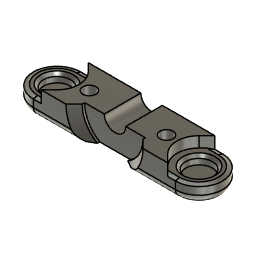
Folding propeller hub v7 (Autodesk Fusion 360 design; units mm, degrees)
Autodesk Fusion 360 part; units mm, degrees
sketch "Sketch1" plane through (0, 0, 0) normal (0, 0, 1) x (1, 0, 0)
  line L0 (-17.5, 0) -> (17.5, 0) construction
  circle A0 centre (-17.5, 0) radius 3.3
  circle A1 centre (17.5, 0) radius 3.3
  arc A2 (-17.5, 5.8) -> (-17.5, -5.8) centre (-17.5, 0) ccw
  line L1 (0, 5.8) -> (0, -5.8) construction
  arc A3 (17.5, -5.8) -> (17.5, 5.8) centre (17.5, 0) ccw
  circle A4 centre (-17.5, 0) radius 5.45
  line L2 (-17.5, 5.8) -> (17.5, 5.8)
  line L3 (17.5, -5.8) -> (-17.5, -5.8)
  line L4 (-13.6463, 3.8537) -> (-15.5925, 5.8)
  line L5 (-13.6463, -3.8537) -> (-15.5925, -5.8)
  line L6 (13.6463, 3.8537) -> (15.5925, 5.8)
  circle A5 centre (17.5, 0) radius 5.45
  line L7 (-2.5, 5.8) -> (-2.5, -5.8) construction
  line L8 (2.5, 5.8) -> (2.5, -5.8) construction
  circle A6 centre (-9.5, 0) radius 1.625
  circle A7 centre (9.5, 0) radius 1.625
  line L9 (13.6463, -3.8537) -> (15.5925, -5.8)
  dimension "d1" = 6.6
  dimension "d2" = 35
  dimension "d3" = 2.5
  dimension "d4" = 10.9
  dimension "d5" = 45
  dimension "d6" = 5
  dimension "d7" = 3.25
  dimension "d8" = 19
  dimension "d33" = 45
  constraint horizontal L0
  constraint midpoint origin L0
  constraint coincident L0.start A0.centre
  constraint coincident L0.end A1.centre
  constraint equal A0 A1
  constraint perpendicular L0 L1
  constraint symmetric A2 L1 A3
  constraint coincident origin L1
  constraint concentric A0 A4
  constraint tangent A3 L2
  constraint tangent A2 L2
  constraint tangent A2 L3
  constraint tangent A3 L3
  constraint midpoint L1.start L2
  constraint midpoint L1.end L3
  constraint coincident A4 L4.start
  constraint coincident L2 L4.end
  constraint tangent A4 L4
  constraint coincident A4 L5.start
  constraint coincident L3 L5.end
  constraint symmetric L1 A4 A5
  constraint symmetric L1 L4.start L6.start
  constraint symmetric L1 L4.end L6.end
  constraint coincident L2 L7.start
  constraint coincident L3 L7.end
  constraint perpendicular L3 L7
  constraint coincident L2 L8.start
  constraint coincident L3 L8.end
  constraint perpendicular L3 L8
  constraint coincident L0 A6.centre
  constraint coincident L0 A7.centre
  constraint symmetric L1 A6 A7
  constraint tangent A4 L5
  constraint symmetric L1 L5.start L9.start
  constraint symmetric L1 L5.end L9.end
  measures "d1" diameter of A0
  measures "d2" distance of L0.start L0.end
  measures "d3" distance of A0 A2
  measures "d4" diameter of A4
  measures "d5" angle of L2 L4
  measures "d6" distance of L7 L8
  measures "d7" diameter of A6
  measures "d8" distance of A6.centre A7.centre
  measures "d33" angle of L3 L5
extrude "Extrude1" add sketch "Sketch1" along normal mid plane 13 contours A0 | A1 | A2 A4 L2 L3 L4 L5 | A4 L2 L3 L4 L5 L6 A5 L9 | A3 L2 L3 L6 A5 L9 | A4 | A5 makes body 1
extrude "Extrude2" cut sketch "Sketch1" along normal mid plane 5.25 contours A0 | A1 | A2 A4 L2 L3 L4 L5 | A3 L2 L3 L6 A5 L9 | A4 | A5 bodies 1
extrude "Extrude3" cut sketch "Sketch1" along normal mid plane 9.4 contours A0 | A1 bodies 1
chamfer "Chamfer1" distance 0.7 angle 45 4 edges at (14.4233, -1.1933, 2.625) (14.4233, 1.1933, -2.625) (-20.5767, -1.1933, 2.625) (-20.5767, 1.1933, -2.625) on bodies 1
sketch "Sketch2" plane through (0, -5.8, 0) normal (0, -1, 0) x (1, 0, 0)
  line L0 (17.5, -6.5) -> (17.5, -2.625)
  line L1 (-15.5925, -2.625) -> (-17.5, -2.625)
  line L2 (17.5, 2.625) -> (17.5, 6.5)
  line L3 (-17.5, -2.625) -> (-17.5, -6.5)
  line L4 (-17.5, 2.625) -> (-15.5925, 2.625)
  circle A0 centre (0, 0) radius 2.65
  circle A1 centre (0, 0) radius 7.5
  line L5 (-17.5, -6.5) -> (17.5, -6.5)
  line L6 (17.5, 6.5) -> (-17.5, 6.5)
  line L7 (-17.5, 6.5) -> (-17.5, 2.625)
  line L8 (-15.5925, 2.625) -> (-15.5925, -2.625)
  line L9 (17.5, -2.625) -> (15.5925, -2.625)
  line L10 (15.5925, -2.625) -> (15.5925, 2.625)
  line L11 (15.5925, 2.625) -> (17.5, 2.625)
  dimension "d18" = 5.3
  dimension "d25" = 15
  constraint coincident A0.centre A1.centre
  constraint concentric A0 A1
  measures "d18" diameter of A0
  measures "d25" diameter of A1
extrude "Extrude4" cut sketch "Sketch2" against normal up to surface (11.6 mm away) contours A0 bodies 1
extrude "Extrude5" cut sketch "Sketch2" along normal up to surface (2.6 mm away) from surface at -2.6 contours A1 L5 L6 | A1 L5 | A1 L6 | A0 bodies 1
chamfer "Chamfer3" distance 2 angle 45 2 edges at (-7.5, -5.8, 0) (7.5, -5.8, 0) measured on face at (-12.895, -5.8, 0) measured on face at (12.895, -5.8, 0) on bodies 1
chamfer "Chamfer2" distance 1 angle 30 10 edges at (0, 5.8, -6.5) (23.3, 0, -6.5) (-12.2141, -5.8, -6.5) (12.2141, -5.8, -6.5) (-23.3, 0, -6.5) (0, 5.8, 6.5) (-23.3, 0, 6.5) (12.2141, -5.8, 6.5) (-12.2141, -5.8, 6.5) (23.3, 0, 6.5) measured on face at (-15.375, 0, -6.5) measured on face at (-15.375, 0, -6.5) measured on face at (-15.375, 0, -6.5) measured on face at (-15.375, 0, -6.5) measured on face at (-15.375, 0, -6.5) measured on face at (-15.375, 0, 6.5) measured on face at (-15.375, 0, 6.5) measured on face at (-15.375, 0, 6.5) measured on face at (-15.375, 0, 6.5) measured on face at (-15.375, 0, 6.5) on bodies 1
fillet "Fillet2" radius 2 10 edges at (-12.4639, -5.8, 5.9226) (12.4639, -5.8, 5.9226) (23.3, 0, 5.9226) (0, 5.8, 5.9226) (-23.3, 0, 5.9226) (12.4639, -5.8, -5.9226) (-12.4639, -5.8, -5.9226) (-23.3, 0, -5.9226) (0, 5.8, -5.9226) (23.3, 0, -5.9226) on bodies 1
chamfer "Chamfer4" distance 0.3 distance2 1 13 edges at (23.3, 0, -2.625) (16.5463, -5.8, -2.625) (16.5463, 5.8, -2.625) (23.3, 0, 2.625) (16.5463, 5.8, 2.625) (-16.5463, -5.8, 2.625) (16.5463, -5.8, 2.625) (-23.3, 0, -2.625) (-16.5463, 5.8, -2.625) (-16.5463, -5.8, -2.625) (-23.3, 0, 2.625) (-16.5463, -5.8, 2.625) (-16.5463, 5.8, 2.625) measured on face at (22.7219, -2.5243, -3.3394) measured on face at (13.5617, -5.8, 0) measured on face at (11.2784, 5.8, 0) measured on face at (22.7219, 2.5243, 3.3394) measured on face at (11.2784, 5.8, 0) measured on face at (-13.5617, -5.8, 0) measured on face at (13.5617, -5.8, 0) measured on face at (-22.7219, 2.5243, -3.3394) measured on face at (11.2784, 5.8, 0) measured on face at (-13.5617, -5.8, 0) measured on face at (-22.7219, -2.5243, 3.3394) measured on face at (-13.5617, -5.8, 0) measured on face at (11.2784, 5.8, 0) on bodies 1
split "Split1" by plane through (0, 0, 0) normal (0, 0, 1) bodies 1 makes body 2 at (-15.375, 0, 6.5)
hidden bodies 2
equation "d9 = 9 mm + 4 mm"
named bodies: "Folding prop hub"
